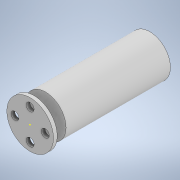
# Autodesk Inventor part: Cylinder
Saved by Autodesk Inventor 2022 (Build 260153000, 153)
## iProperties
Created: 2022-03-08
Part Number: Cylinder
Material: Generic
Document SubType Name: Modeling
Designer: karee
Density: 1 g/cm^3
Appearance: Default
Author: karee
Autodesk Inventor part; units mm, degrees
ref_plane "YZ Plane" through (0, 0, 0) normal (1, 0, 0) x (0, 1, 0)
ref_plane "XZ Plane" through (0, 0, 0) normal (0, 1, 0) x (-1, 0, 0)
ref_plane "XY Plane" through (0, 0, 0) normal (0, 0, 1) x (1, 0, 0)
sketch "Sketch1" plane through (0, 0, 0) normal (0, 0, 1) x (1, 0, 0)
  circle A0 centre (0, 0) radius 2.8166
  constraints: 1 centre point, 1 coincident
extrude "Extrusion1" add sketch "Sketch1" along normal blind 14.2875
sketch "Sketch2" plane through (0, 0, 14.2875) normal (0, 0, 1) x (1, 0, 0)
  circle A0 centre (0, 0) radius 0.8892
  constraints: 1 centre point, 1 coincident
extrude "Extrusion2" add sketch "Sketch2" along normal blind 1.5875
sketch "Sketch3" plane through (0, 0, 15.875) normal (0, 0, 1) x (1, 0, 0)
  circle A0 centre (0, 0) radius 3.1943
  constraints: 1 centre point, 1 coincident
extrude "Extrusion3" add sketch "Sketch3" along normal blind 0.508
sketch "Sketch4" plane through (0, 0, 16.383) normal (0, 0, 1) x (1, 0, 0)
  point P0 (0, 0)
sketch "Sketch5" plane through (0, 0, 16.383) normal (0, 0, 1) x (1, 0, 0)
  circle A0 centre (0, 0) radius 3.1943
  circle A1 centre (2.0744, 0) radius 0.5486
  circle A2 centre (0, -2.0828) radius 0.5461
  circle A3 centre (-2.0828, 0) radius 0.5461
  circle A4 centre (0, 2.0828) radius 0.5461
  constraints: 5 centre point, 1 coincident
extrude "Extrusion4" cut sketch "Sketch5" against normal blind 0.508 contours A1 | A2 | A3 | A4
sketch "Sketch6" plane through (0, 0, 16.383) normal (0, 0, 1) x (1, 0, 0)
  point P0 (0, 0)
body "Solid1"
